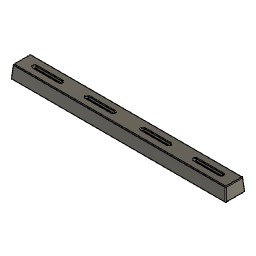
Bed (Autodesk Fusion 360 design; units mm, degrees)
Autodesk Fusion 360 part; units mm, degrees
ref_plane "WorkPlane1" through (0, 0, 38.1) normal (0, 0, 1) x (1, 0, 0)
sketch "Top" plane through (0, 0, 0) normal (0, 0, 1) x (1, 0, 0) in component "Ways"
  line L0 (622.3, 53.975, 38.1) -> (3.175, 53.975, 38.1)
  line L1 (3.175, 53.975, 38.1) -> (3.175, 3.175, 38.1)
  line L2 (622.3, 3.175, 38.1) -> (622.3, 53.975, 38.1)
  line L3 (3.175, 3.175, 38.1) -> (622.3, 3.175, 38.1)
sketch "Bottom" plane through (0, 0, 0) normal (0, 0, 1) x (1, 0, 0) in component "Ways"
  line L0 (0, 0) -> (625.475, 0)
  line L1 (625.475, 0) -> (625.475, 57.15)
  line L2 (625.475, 57.15) -> (0, 57.15)
  line L3 (0, 57.15) -> (0, 0)
  line L4 (6.35, 6.35) -> (619.125, 6.35)
  line L5 (619.125, 6.35) -> (619.125, 50.8)
  line L6 (619.125, 50.8) -> (6.35, 50.8)
  line L7 (6.35, 50.8) -> (6.35, 6.35)
  line L8 (156.3688, 50.8) -> (156.3688, 6.35)
  line L9 (161.1312, 6.35) -> (161.1312, 50.8)
  line L10 (307.1812, 50.8) -> (307.1812, 6.35)
  line L11 (311.9437, 6.35) -> (311.9437, 50.8)
  line L12 (464.3437, 50.8) -> (464.3437, 6.35)
  line L13 (469.1062, 6.35) -> (469.1062, 50.8)
  dimension "d1" = 625.475
  dimension "d2" = 57.15
  dimension "d5" = -6.35
  constraint horizontal L0
  constraint vertical L1
  constraint horizontal L2
  constraint vertical L3
  constraint coincident L0.start L3.end
  constraint coincident L6 L8.start
  constraint coincident L4 L8.end
  constraint perpendicular L4 L8
  constraint coincident L4 L9.start
  constraint coincident L6 L9.end
  constraint perpendicular L6 L9
  constraint coincident L6 L10.start
  constraint coincident L4 L10.end
  constraint perpendicular L4 L10
  constraint coincident L4 L11.start
  constraint coincident L6 L11.end
  constraint perpendicular L6 L11
  constraint coincident L6 L12.start
  constraint coincident L4 L12.end
  constraint perpendicular L4 L12
  constraint coincident L4 L13.start
  constraint coincident L6 L13.end
  constraint perpendicular L6 L13
  measures "d1" distance of L0.start L0.end
  measures "d2" distance of L0.start L2.end
sketch "Middle" plane through (0, 0, 0) normal (0, 0, 1) x (1, 0, 0) in component "Ways"
  line L0 (615.95, 47.625, 31.75) -> (9.525, 47.625, 31.75)
  line L1 (615.95, 9.525, 31.75) -> (615.95, 47.625, 31.75)
  line L2 (9.525, 9.525, 31.75) -> (615.95, 9.525, 31.75)
  line L3 (9.525, 47.625, 31.75) -> (9.525, 9.525, 31.75)
loft "Loft1" add profiles "Bottom", "Top" section 1 section 2 contours L0 L1 L2 L3 in plane through (0, 0, 38.1) normal (0, 0, 1) makes body 1 in component "Ways"
loft "Loft2" cut profiles "Bottom", "Middle" section 1 contours L4 L6 L7 L8 | L4 L6 L8 L9 | L4 L6 L9 L10 | L4 L6 L10 L11 | L4 L6 L11 L12 | L4 L6 L12 L13 | L4 L5 L6 L13 section 2 contours L0 L1 L2 L3 in plane through (0, 0, 31.75) normal (0, 0, 1) bodies 1 in component "Ways"
sketch "Holes" plane through (0, 0, 38.1) normal (0, 0, 1) x (1, 0, 0) in component "Ways"
  line L0 (3.175, 3.175) -> (622.3, 3.175)
  line L1 (622.3, 3.175) -> (622.3, 53.975)
  line L2 (622.3, 53.975) -> (3.175, 53.975)
  line L3 (3.175, 53.975) -> (3.175, 3.175)
  arc A0 (41.275, 33.3375) -> (41.275, 23.8125) centre (41.275, 28.575) ccw
  arc A1 (117.475, 23.8125) -> (117.475, 33.3375) centre (117.475, 28.575) ccw
  line L4 (117.475, 23.8125) -> (41.275, 23.8125)
  line L5 (41.275, 33.3375) -> (117.475, 33.3375)
  arc A2 (193.675, 33.3375) -> (193.675, 23.8125) centre (193.675, 28.575) ccw
  arc A3 (269.875, 23.8125) -> (269.875, 33.3375) centre (269.875, 28.575) ccw
  line L6 (193.675, 33.3375) -> (269.875, 33.3375)
  line L7 (269.875, 23.8125) -> (193.675, 23.8125)
  line L8 (584.2, 23.8125) -> (508, 23.8125)
  line L9 (431.8, 23.8125) -> (355.6, 23.8125)
  line L10 (355.6, 33.3375) -> (431.8, 33.3375)
  line L11 (508, 33.3375) -> (584.2, 33.3375)
  arc A4 (355.6, 33.3375) -> (355.6, 23.8125) centre (355.6, 28.575) ccw
  arc A5 (431.8, 23.8125) -> (431.8, 33.3375) centre (431.8, 28.575) ccw
  arc A6 (508, 33.3375) -> (508, 23.8125) centre (508, 28.575) ccw
  arc A7 (584.2, 23.8125) -> (584.2, 33.3375) centre (584.2, 28.575) ccw
  line L12 (155.575, 53.975) -> (155.575, 3.175)
  line L13 (161.925, 53.975) -> (161.925, 3.175)
  line L14 (306.3875, 53.975) -> (306.3875, 3.175)
  line L15 (312.7375, 53.975) -> (312.7375, 3.175)
  line L16 (463.55, 53.975) -> (463.55, 3.175)
  line L17 (469.9, 53.975) -> (469.9, 3.175)
  dimension "d33" = 9.525
  dimension "d34" = 9.525
  dimension "d35" = 9.525
  dimension "d36" = 9.525
  dimension "d37" = 9.525
  dimension "d38" = 9.525
  dimension "d39" = 9.525
  dimension "d40" = 9.525
  dimension "d41" = 76.2
  dimension "d42" = 76.2
  dimension "d43" = 76.2
  dimension "d44" = 76.2
  constraint perpendicular L1 L5
  constraint perpendicular L3 L8
  constraint coincident A1.start L8
  constraint collinear L4 L8
  constraint collinear L5 L6
  constraint collinear L6 L10
  constraint collinear L7 L8
  constraint collinear L8 L9
  constraint collinear L10 L11
  constraint coincident L2 L12.start
  constraint coincident L0 L12.end
  constraint perpendicular L0 L12
  constraint coincident L2 L13.start
  constraint coincident L0 L13.end
  constraint perpendicular L0 L13
  constraint coincident L2 L14.start
  constraint coincident L0 L14.end
  constraint perpendicular L0 L14
  constraint coincident L2 L15.start
  constraint coincident L0 L15.end
  constraint perpendicular L0 L15
  constraint coincident L2 L16.start
  constraint coincident L0 L16.end
  constraint perpendicular L0 L16
  constraint coincident L2 L17.start
  constraint coincident L0 L17.end
  constraint perpendicular L0 L17
  measures "d33" diameter of A0
  measures "d34" diameter of A1
  measures "d35" diameter of A2
  measures "d36" diameter of A3
  measures "d37" diameter of A7
  measures "d38" diameter of A6
  measures "d39" diameter of A5
  measures "d40" diameter of A4
  measures "d41" distance of A0.centre A1.centre
  measures "d42" distance of A2.centre A3.centre
  measures "d43" distance of A5.centre A4.centre
  measures "d44" distance of A7.centre A6.centre
extrude "Extrude1" cut sketch "Holes" against normal up to surface (6.35 mm away) draft -14 contours A0 A1 L4 L5 | A2 A3 L6 L7 | L8 L11 A6 A7 | L9 L10 A4 A5 bodies 1 in component "Ways"
copy_body "CutPasteBodies1" bodies 1 removing the originals makes body 2 in component "Ways"
fillet "Fillet1" radius 2 5 faces at (14.2991, 28.7664, 38.1) (209.55, 1.0583, 12.7) (624.4167, 20.1083, 12.7) (209.55, 56.0917, 12.7) (1.0583, 37.0417, 12.7) on bodies 2 in component "Ways"
ref_plane "WorkPlane1" through (0, 0, 38.1) normal (0, 0, 1) x (1, 0, 0) in component "Ways"
loft "Loft1'" add profiles "Bottom", "Holes" section 1 contours L4 L6 L8 L9 section 2 contours L0 L2 L12 L13 separate body makes body 3 in component "Ways"
loft "Loft2'" add profiles "Bottom", "Holes" section 1 contours L4 L6 L10 L11 section 2 contours L0 L2 L14 L15 separate body makes body 4 in component "Ways"
loft "Loft3" add profiles "Bottom", "Holes" section 1 contours L4 L6 L12 L13 section 2 contours L0 L2 L16 L17 separate body makes body 5 in component "Ways"
fillet "Fillet2" radius 2 1 faces at (467.7833, 37.0417, 38.1) on bodies 5 in component "Ways"
fillet "Fillet3" radius 2 1 faces at (308.5042, 37.0417, 38.1) on bodies 4 in component "Ways"
fillet "Fillet4" radius 2 1 faces at (157.6917, 37.0417, 38.1) on bodies 3 in component "Ways"
fillet "Fillet5" radius 2 2 edges at (156.3688, 28.575, 0) (161.1313, 28.575, 0) on bodies 3 in component "Ways"
fillet "Fillet6" radius 2 2 edges at (307.1812, 28.575, 0) (311.9437, 28.575, 0) on bodies 4 in component "Ways"
fillet "Fillet7" radius 2 2 edges at (464.3437, 28.575, 0) (469.1062, 28.575, 0) on bodies 5 in component "Ways"
combine "Combine1" operation add target body 2 tool bodies 3 4 5 in component "Ways"
component "Ways" placed x (1, 0, 0) y (0, 1, 0) z (0, 0, 1) at (0, 0, 0)
component "Mounting Bases" placed x (1, 0, 0) y (0, 1, 0) z (0, 0, 1) at (0, 0, 0) in component "Ways"
